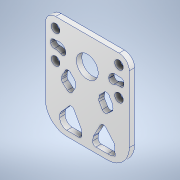
# Autodesk Inventor part: CaseSheet
Saved by Autodesk Inventor 2020.2 (Build 242310000, 310)
## iProperties
Created: 2020-01-19
Part Number: CaseSheet
Material: Aluminum 6061
Document SubType Name: Sheet Metal
Designer: Paul Lefeuvre
Density: 2.7 g/cm^3
Appearance: Aluminum - Flat
Mass: 66.3516 g
Surface Area: 151.342 cm^2
Volume: 24.5747 cm^3
Sheet Metal Rule: Default_mm
Author: Paul Lefeuvre
Autodesk Inventor part; units mm, degrees
ref_plane "YZ Plane" through (0, 0, 0) normal (1, 0, 0) x (0, 1, 0)
ref_plane "XZ Plane" through (0, 0, 0) normal (0, 1, 0) x (-1, 0, 0)
ref_plane "XY Plane" through (0, 0, 0) normal (0, 0, 1) x (1, 0, 0)
sketch "Sketch1" plane through (0, 0, 0) normal (0, 0, 1) x (1, 0, 0)
  circle A0 centre (0, 0) radius 20.6375 construction
  line L0 (-6.35, 3.6662) -> (0, 7.3323) construction
  line L1 (0, 7.3323) -> (6.35, 3.6662) construction
  line L2 (6.35, 3.6662) -> (6.35, -3.6662) construction
  line L3 (6.35, -3.6662) -> (0, -7.3323) construction
  line L4 (0, -7.3323) -> (-6.35, -3.6662) construction
  line L5 (-6.35, -3.6662) -> (-6.35, 3.6662) construction
  line L6 (0, 0) -> (0, 22.8196) construction
  line L7 (38.941, 16.1375) -> (38.941, -45.6375)
  line L8 (18.941, -65.6375) -> (-36.941, -65.6375)
  circle A1 centre (29.441, 16.1375) radius 3 construction
  circle A2 centre (29.441, 16.1375) radius 7.5 construction
  line L9 (-38.941, 16.1375) -> (-38.941, -63.6375)
  circle A3 centre (29.441, 16.1375) radius 9.5
  line L10 (29.441, 25.6375) -> (-29.441, 25.6375)
  circle A4 centre (-29.441, 16.1375) radius 3 construction
  circle A5 centre (-29.441, 16.1375) radius 9.5
  circle A6 centre (29.441, 16.1375) radius 4
  circle A7 centre (-29.441, 16.1375) radius 4
  circle A8 centre (-29.441, -10.1375) radius 3 construction
  circle A9 centre (-29.441, -10.1375) radius 10.5 construction
  circle A10 centre (-29.441, -10.1375) radius 4
  line L11 (0, -20.6375) -> (-54.2194, -20.6375) construction
  arc A11 (18.941, -65.6375) -> (38.941, -45.6375) centre (18.941, -45.6375) ccw
  circle A12 centre (0, 0) radius 7.5 construction
  arc A13 (-38.941, -63.6375) -> (-36.941, -65.6375) centre (-36.941, -63.6375) ccw
  circle A14 centre (0, 0) radius 9.5 construction
  circle A15 centre (0, 0) radius 10.1
  circle A16 centre (-29.441, -10.1375) radius 7.5 construction
  circle A17 centre (-29.441, 16.1375) radius 7.5 construction
  circle A18 centre (-29.441, -10.1375) radius 9.5 construction
  circle A19 centre (29.441, -10.1375) radius 3 construction
  circle A20 centre (29.441, -10.1375) radius 7.5 construction
  circle A21 centre (29.441, -10.1375) radius 10.5 construction
  circle A22 centre (29.441, -10.1375) radius 9.5 construction
  circle A23 centre (29.441, -10.1375) radius 4
  dimension "d0" = 41.275
  dimension "d1" = 12.7
  dimension "d3" = 65.6375
  dimension "d4" = 6
  dimension "d6" = 15
  dimension "d7" = 2
  dimension "d9" = 6
  dimension "d12" = 1
  dimension "d13" = 1
  dimension "d14" = 6
  dimension "d18" = 1
  dimension "d19" = 20
  dimension "d20" = 15
  dimension "d21" = 2
  dimension "d22" = 19
  dimension "d23" = 0.6
  dimension "d26" = 15
  dimension "d27" = 3
  dimension "d29" = 2
  dimension "d30" = 15
  dimension "d31" = 2
  dimension "d37" = 6
  dimension "d38" = 15
  dimension "d39" = 3
  dimension "d40" = 2
  dimension "d41" = 1
  dimension "d42" = 25.6375
  constraints: 24 end point, 23 centre point, 12 tangent, 10 coincident, 8 point on circle, 4 horizontal, 2 vertical, 1 perpendicular, 1 point on line, 1 vertical alignment, 17 other
  measures "d1" distance of L0.start L1.end
  measures "d3" distance from line of point (0, 0) L8
  measures "d4" diameter of A1
  measures "d6" diameter of A2
  measures "d7" radial gap between concentric circles of A2 A3
  measures "d9" diameter of A4
  measures "d12" radial gap between concentric circles of A1 A6
  measures "d13" radial gap between concentric circles of A4 A7
  measures "d14" diameter of A8
  measures "d18" radial gap between concentric circles of A8 A10
  measures "d19" radius of A11
  measures "d20" diameter of A12
  measures "d21" radius of A13
  measures "d22" diameter of A14
  measures "d23" radial gap between concentric circles of A14 A15
  measures "d26" diameter of A16
  measures "d27" radial gap between concentric circles of A9 A16
  measures "d29" radial gap between concentric circles of A5 A17
  measures "d30" diameter of A17
  measures "d31" radial gap between concentric circles of A16 A18
  measures "d37" diameter of A19
  measures "d38" diameter of A20
  measures "d39" radial gap between concentric circles of A20 A21
  measures "d40" radial gap between concentric circles of A20 A22
  measures "d41" radial gap between concentric circles of A19 A23
  measures "d42" distance from line of L10 point (0, 0)
extrude "Extrusion1" add sketch "Sketch1" along normal blind 5
sketch "Sketch2" plane through (0, 0, 5) normal (0, 0, 1) x (1, 0, 0)
  circle A0 centre (0, 0) radius 20
  circle A1 centre (29.441, 16.1375) radius 4 projected
  circle A2 centre (29.441, 16.1375) radius 9.5
  circle A3 centre (29.441, -10.1375) radius 9.5
  circle A4 centre (-29.441, 16.1375) radius 9.5
  circle A5 centre (-29.441, -10.1375) radius 9.5
  circle A6 centre (29.441, 16.1375) radius 4 projected
  circle A7 centre (-29.441, 16.1375) radius 4 projected
  circle A8 centre (-29.441, -10.1375) radius 4 projected
  circle A9 centre (29.441, -10.1375) radius 4 projected
  arc A10 (-19.9843, 0.7915) -> (-27.3195, 6.8774) centre (-25.9796, 1.0289) ccw
  arc A11 (-20.4937, 19.3304) -> (-11.4175, 16.4208) centre (-14.8427, 21.347) ccw
  arc A12 (-24.5405, -1.9991) -> (-19.9938, 0.4965) centre (-22.9929, 0.571) ccw
  arc A13 (-15.4496, -12.7008) -> (-20.5688, -13.5335) centre (-17.767, -14.6059) ccw
  arc A14 (20.5688, -13.5335) -> (15.4496, -12.7008) centre (17.767, -14.6059) ccw
  arc A15 (19.9938, 0.4965) -> (24.5405, -1.9991) centre (22.9929, 0.571) ccw
  arc A16 (27.3195, 6.8774) -> (19.9843, 0.7915) centre (25.9796, 1.0289) ccw
  arc A17 (11.4175, 16.4208) -> (20.4937, 19.3304) centre (14.8427, 21.347) ccw
  arc A18 (-29.441, 25.6375) -> (-38.941, 16.1375) centre (-29.441, 16.1375) ccw projected
  line L0 (29.441, 25.6375) -> (-29.441, 25.6375)
  line L1 (-38.941, 16.1375) -> (-38.941, -10.1375)
  line L2 (38.941, -45.6375) -> (38.941, 16.1375) projected
  line L3 (38.941, -10.1375) -> (38.941, 16.1375)
  line L4 (33.941, -1.7709) -> (33.941, 7.7709)
  line L5 (21.0744, 20.6375) -> (-21.0744, 20.6375)
  line L6 (-33.941, 7.7709) -> (-33.941, -1.7709)
  line L7 (29.3892, -56.146) -> (36.456, -16.5438)
  line L8 (-29.3891, -56.1463) -> (-36.456, -16.5438)
  line L9 (0, 40.0952) -> (0, -100.5638) construction
  line L10 (-33.941, -30.6375) -> (-33.941, -60.6375)
  line L11 (7.9638, -60.6375) -> (33.941, -60.6375)
  line L12 (33.941, -60.6375) -> (33.941, -30.6375)
  line L13 (-38.941, 16.1375) -> (-38.941, -63.6375) projected
  line L14 (-36.941, -65.6375) -> (18.941, -65.6375) projected
  arc A19 (5, -57.1728) -> (7.9638, -60.6375) centre (7.9638, -57.6375) ccw
  arc A20 (-7.9638, -60.6375) -> (-5, -57.1728) centre (-7.9638, -57.6375) ccw
  arc A21 (18.941, -60.6375) -> (33.941, -45.6375) centre (18.941, -45.6375) ccw
  arc A22 (-33.941, -45.6375) -> (-19.0796, -60.6375) centre (-18.9404, -45.6375) ccw
  arc A23 (-11.0678, -18.4694) -> (-12.8408, -15.3334) centre (-16.1319, -19.2633) ccw
  arc A24 (12.4443, -15.6569) -> (11.1641, -17.8551) centre (14.6225, -18.3973) ccw
  arc A25 (23.8228, -21.0563) -> (21.9787, -16.0165) centre (15.2066, -21.3517) ccw
  arc A26 (-22.076, -16.138) -> (-23.7755, -20.5374) centre (-16.1754, -20.9454) ccw
  arc A27 (-25.551, -53.6187) -> (-18.8648, -60.638) centre (-18.8984, -53.9758) ccw
  arc A28 (-32.8608, -51.2269) -> (-30.3932, -50.5194) centre (-31.6635, -50.7461) ccw
  line L15 (-7.9638, -60.6375) -> (-33.941, -60.6375)
  arc A29 (18.941, -65.6375) -> (38.941, -45.6375) centre (18.941, -45.6375) ccw projected
  arc A30 (-38.941, -45.6375) -> (-18.941, -65.6375) centre (-18.941, -45.6375) ccw
  line L16 (-18.941, -65.6375) -> (-38.941, -65.6375)
  line L17 (-38.941, -65.6375) -> (-38.941, -45.6375)
  line L18 (-22.8299, -24.4834) -> (-18.4556, -28.2868)
  line L19 (-12.5756, -34.6041) -> (-11.985, -35.0783)
  line L20 (-11.0833, -22.6011) -> (-13.8809, -27.5086)
  line L21 (-20.734, -34.9273) -> (-21.3309, -35.346)
  line L22 (-21.3531, -31.2513) -> (-20.7979, -31.6097)
  line L23 (-12.2684, -40.7606) -> (-5.9104, -52.4836)
  line L24 (-12.1247, -31.1196) -> (-12.5828, -31.4909)
  line L25 (-17.173, -40.2264) -> (-24.665, -48.8747)
  line L26 (-11.3855, -16.4429) -> (-10.7258, -20.6508)
  line L27 (-23.8571, -22.0587) -> (-23.6203, -17.6454)
  line L28 (-25.8376, -58.9584) -> (-25.3932, -50.6782)
  line L29 (-24.4767, -33.6015) -> (-24.435, -32.8244)
  line L30 (-8.8895, -32.3636) -> (-8.757, -33.209)
  line L31 (-5.5838, -53.4492) -> (-5, -57.1728)
  arc A31 (-12.5828, -31.4909) -> (-12.5756, -34.6041) centre (-11.3234, -33.0446) ccw
  arc A32 (-20.734, -34.9273) -> (-20.7979, -31.6097) centre (-21.8827, -33.29) ccw
  arc A33 (-18.4556, -28.2868) -> (-13.8809, -27.5086) centre (-16.4871, -26.0229) ccw
  arc A34 (-12.2684, -40.7606) -> (-17.173, -40.2264) centre (-14.9055, -42.1908) ccw
  arc A35 (-23.8571, -22.0587) -> (-22.8299, -24.4834) centre (-20.8614, -22.2195) ccw
  arc A36 (-11.0833, -22.6011) -> (-10.7258, -20.6508) centre (-13.6896, -21.1154) ccw
  arc A37 (-24.665, -48.8747) -> (-25.3932, -50.6782) centre (-22.3975, -50.839) ccw
  arc A38 (-5.5838, -53.4492) -> (-5.9104, -52.4836) centre (-8.5476, -53.9139) ccw
  line L32 (22.8299, -24.4834) -> (18.4556, -28.2868)
  line L33 (11.0833, -22.6011) -> (13.8809, -27.5086)
  line L34 (12.2684, -40.7606) -> (5.9104, -52.4836)
  line L35 (17.173, -40.2264) -> (24.665, -48.8747)
  arc A39 (13.8809, -27.5086) -> (18.4556, -28.2868) centre (16.4871, -26.0229) ccw
  arc A40 (17.173, -40.2264) -> (12.2684, -40.7606) centre (14.9055, -42.1908) ccw
  arc A41 (22.8299, -24.4834) -> (23.8571, -22.0587) centre (20.8614, -22.2195) ccw
  arc A42 (10.7258, -20.6508) -> (11.0833, -22.6011) centre (13.6896, -21.1154) ccw
  arc A43 (25.3932, -50.6782) -> (24.665, -48.8747) centre (22.3975, -50.839) ccw
  arc A44 (5.9104, -52.4836) -> (5.5838, -53.4492) centre (8.5476, -53.9139) ccw
  line L36 (10.7258, -20.6508) -> (11.3855, -16.4429)
  line L37 (23.7081, -17.7127) -> (23.8571, -22.0587)
  line L38 (5, -57.1728) -> (5.5838, -53.4492)
  line L39 (25.3932, -50.6782) -> (25.8319, -58.961)
  arc A45 (30.3932, -50.5194) -> (32.8608, -51.2269) centre (31.6635, -50.7461) ccw
  arc A46 (-21.3531, -31.2513) -> (-24.435, -32.8244) centre (-22.4378, -32.9316) ccw
  arc A47 (-24.4767, -33.6015) -> (-21.3309, -35.346) centre (-22.4795, -33.7087) ccw
  arc A48 (-11.985, -35.0783) -> (-8.757, -33.209) centre (-10.7328, -33.5188) ccw
  arc A49 (-8.8895, -32.3636) -> (-12.1247, -31.1196) centre (-10.8654, -32.6733) ccw
  line L40 (12.5756, -34.6041) -> (11.985, -35.0783)
  line L41 (20.734, -34.9273) -> (21.3309, -35.346)
  line L42 (21.3531, -31.2513) -> (20.7979, -31.6097)
  line L43 (12.1247, -31.1196) -> (12.5828, -31.4909)
  line L44 (24.4767, -33.6015) -> (24.435, -32.8244)
  line L45 (8.8895, -32.3636) -> (8.757, -33.209)
  arc A50 (12.5756, -34.6041) -> (12.5828, -31.4909) centre (11.3234, -33.0446) ccw
  arc A51 (20.7979, -31.6097) -> (20.734, -34.9273) centre (21.8827, -33.29) ccw
  arc A52 (24.435, -32.8244) -> (21.3531, -31.2513) centre (22.4378, -32.9316) ccw
  arc A53 (21.3309, -35.346) -> (24.4767, -33.6015) centre (22.4795, -33.7087) ccw
  arc A54 (8.757, -33.209) -> (11.985, -35.0783) centre (10.7328, -33.5188) ccw
  arc A55 (12.1247, -31.1196) -> (8.8895, -32.3636) centre (10.8654, -32.6733) ccw
  arc A56 (-33.941, 2.2722) -> (-30.581, -0.7061) centre (-30.941, 2.2722) ccw
  arc A57 (-30.581, 6.7061) -> (-33.941, 3.7278) centre (-30.941, 3.7278) ccw
  arc A58 (33.941, 3.7278) -> (30.581, 6.7061) centre (30.941, 3.7278) ccw
  arc A59 (30.581, -0.7061) -> (33.941, 2.2722) centre (30.941, 2.2722) ccw
  point P0 (0, -85.153)
  point P1 (-28.5877, -60.6375)
  point P2 (28.5877, -60.6375)
  point P3 (-3.8827, -61.6103)
  point P4 (-24.697, -37.7075)
  point P5 (-9.4273, -28.9333)
  point P6 (-7.9569, -38.3124)
  point P7 (-24.2501, -29.381)
  point P8 (30.3932, -50.5194)
  point P9 (32.8565, -51.2375)
  point P10 (-18.9832, -60.6375)
  dimension "d43" = 40
  dimension "d44" = 6
  dimension "d45" = 6
  dimension "d46" = 6
  dimension "d47" = 6
  dimension "d48" = 3
  dimension "d49" = 3
  dimension "d50" = 3
  dimension "d51" = 3
  dimension "d52" = 5
  dimension "d53" = 5
  dimension "d54" = 5
  dimension "d55" = 5
  dimension "d56" = 5
  dimension "d57" = 5
  dimension "d59" = 3
  dimension "d60" = 15
  dimension "d62" = 20
  dimension "d63" = 2
  dimension "d64" = 3
  dimension "d67" = 2
  dimension "d70" = 3
  dimension "d71" = 3
  dimension "d72" = 3
  dimension "d73" = 3
  dimension "d74" = 10
  dimension "d75" = 5
  constraints: 100 point on circle, 87 end point, 58 tangent, 48 centre point, 39 symmetric about line, 31 point on line, 9 equal radius, 5 vertical, 3 parallel, 2 coincident, 2 horizontal, 2 midpoint, 2 perpendicular, 93 other
  measures "d44" radius of A11
  measures "d45" radius of A17
  measures "d46" radius of A10
  measures "d47" radius of A16
  measures "d48" radius of A13
  measures "d49" radius of A12
  measures "d50" radius of A14
  measures "d51" radius of A15
  measures "d52" distance between parallel lines of L3 L4
  measures "d53" distance between parallel lines of L0 L5
  measures "d54" distance between parallel lines of L1 L6
  measures "d55" distance between parallel lines of L13 L10
  measures "d56" distance between parallel lines of L14 L11
  measures "d57" distance between parallel lines of L2 L12
  measures "d59" radius of A20
  measures "d60" radius of A21
  measures "d62" radius of A30
  measures "d63" radius of A31
  measures "d64" radius of A33
  measures "d67" radius of A46
  measures "d70" radius of A56
  measures "d71" radius of A57
  measures "d72" radius of A58
  measures "d73" radius of A59
  measures "d74" distance of L31.end L38.start
  measures "d75" horizontal distance of L28.end A28.end
extrude "Extrusion2" cut sketch "Sketch2" against normal blind 10 contours A0 A16 A2 A58 L4 A59 A3 A15 | A14 A3 A25 L37 A41 L32 A39 L33 A42 L36 A24 A0 | A0 A12 A5 A56 L6 A57 A4 A10 | A23 L26 A36 L20 A33 L18 A35 L27 A26 A5 A13 A0 | L11 A19 L38 A44 L34 A40 L35 A43 L39 A21 | A30 L10 L15 L14 L16 L17 L13 | A30 L15 L10 | A27 L28 A37 L25 A34 L23 A38 L31 A20 L15
body "Solid1"
